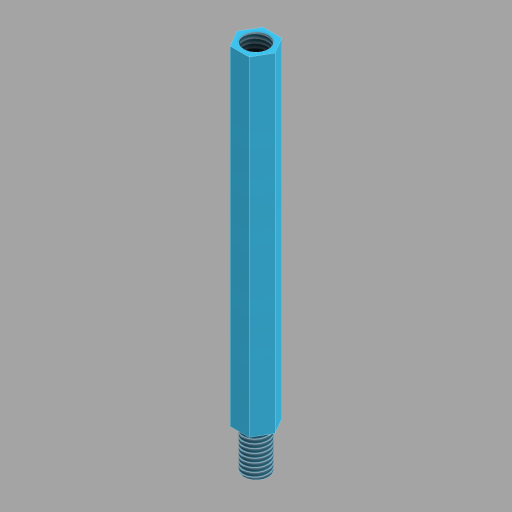
# Autodesk Inventor part: stoyka_M8_80mm
Saved by Autodesk Inventor 2024.2 (Build 282272000, 272)
## iProperties
Created: 2024-01-03
Part Number: stoyka_M8_80mm
Material: Типовые
Document SubType Name: Modeling
Designer: Fedor Orlov
Density: 1 g/cm^3
Appearance: По умолчанию
Author: Fedor Orlov
Autodesk Inventor part; units mm, degrees
ref_plane "YZ Plane" through (0, 0, 0) normal (1, 0, 0) x (0, 1, 0)
ref_plane "XZ Plane" through (0, 0, 0) normal (0, 1, 0) x (-1, 0, 0)
ref_plane "XY Plane" through (0, 0, 0) normal (0, 0, 1) x (1, 0, 0)
sketch "Эскиз1" plane through (0, 0, 0) normal (0, 1, 0) x (-1, 0, 0)
  line L0 (4.6188, 0) -> (2.3094, -4)
  line L1 (2.3094, -4) -> (-2.3094, -4)
  line L2 (-2.3094, -4) -> (-4.6188, 0)
  line L3 (-4.6188, 0) -> (-2.3094, 4)
  line L4 (-2.3094, 4) -> (2.3094, 4)
  line L5 (2.3094, 4) -> (4.6188, 0)
  circle A0 centre (0, 0) radius 3
  dimension "d0" = 8
  dimension "d1" = 8
  dimension "d2" = 6
  constraints: 12 end point, 2 coincident, 1 centre point, 13 other
  measures "d0" distance between parallel lines of L1 L4
  measures "d1" vertical distance of L1.end L4.end
  measures "d2" diameter of A0
extrude "Выдавливание1" add sketch "Эскиз1" along normal blind 80
sketch "Эскиз2" plane through (0, 0, 0) normal (0, -1, 0) x (1, 0, 0)
  circle A0 centre (0, 0) radius 3
  dimension "d5" = 6
  constraints: 1 centre point, 1 coincident
  measures "d5" diameter of A0
extrude "Выдавливание2" add sketch "Эскиз2" along normal blind 10 and the other way blind 10
thread "Резьба2" size "M6x1" class "6g" standard "ANSI Metric M Profile" full length
thread "Резьба3" size "M6x1" class "6H" standard "ANSI Metric M Profile" full length
